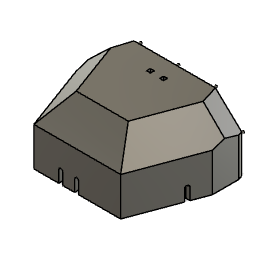
Seismo Case Top S1 v2 (Autodesk Fusion 360 design; units mm, degrees)
Autodesk Fusion 360 part; units mm, degrees
sketch "Sketch1" plane through (0, 0, 0) normal (0, 1, 0) x (1, 0, 0)
  line L0 (-69.1818, 27.2298) -> (-69.1818, -12.7702)
  line L1 (-69.1818, 27.2298) -> (-31.3668, 147.2296)
  line L2 (-31.3668, 147.2296) -> (98.6332, 147.2296)
  line L3 (98.6332, 147.2296) -> (136.3099, 27.1863)
  line L4 (136.3099, 27.1863) -> (136.3099, -12.8137)
  line L5 (136.3099, -12.8137) -> (98.5054, -114.5242)
  line L6 (-69.1818, -12.7702) -> (-31.4946, -114.5242)
  line L7 (-31.4946, -114.5242) -> (98.5054, -114.5242)
  line L8 (-36.0236, 153.5796) -> (103.2956, 153.5796)
  line L9 (103.2956, 153.5796) -> (142.6599, 28.1594)
  line L10 (142.6599, 28.1594) -> (142.6599, -13.9557)
  line L11 (142.6599, -13.9557) -> (102.9196, -120.8742)
  line L12 (102.9196, -120.8742) -> (-35.9143, -120.8742)
  line L13 (-35.9143, -120.8742) -> (-75.5318, -13.9084)
  line L14 (-75.5318, -13.9084) -> (-75.5318, 28.2067)
  line L15 (-75.5318, 28.2067) -> (-36.0236, 153.5796)
  dimension "d1" = 40
  dimension "d2" = 125.817
  dimension "d5" = 125.817
  dimension "d6" = 40
  dimension "d8" = 108.509
  dimension "d10" = 108.509
  dimension "d12" = 162.509
  dimension "d14" = 6.35
  dimension "d15" = 6.35
  dimension "d16" = 6.35
  dimension "d17" = 6.35
  dimension "d18" = 6.35
  dimension "d19" = 6.35
  dimension "d20" = 6.35
  dimension "d21" = 6.35
  dimension "d44" = 130
  dimension "d49" = 130
  constraint vertical L0
  constraint horizontal L2
  constraint vertical L4
  constraint parallel L2 L8
  constraint parallel L3 L9
  constraint perpendicular L8 L10
  constraint parallel L5 L11
  constraint horizontal L12
  constraint vertical L14
  constraint parallel L6 L13
  measures "d1" distance of L0.start L0.end
  measures "d2" distance of L0.start L1.end
  measures "d5" distance of L2.end L3.end
  measures "d6" distance of L3.end L4.end
  measures "d8" distance of L4.end L5.end
  measures "d10" distance of L0.end L6.end
  measures "d12" angle of L14 L15
  measures "d14" distance of L5 L11
  measures "d15" distance of L4 L10
  measures "d16" distance of L3 L9
  measures "d17" distance of L2 L8
  measures "d18" distance of L1 L15
  measures "d19" distance of L0 L14
  measures "d20" distance of L6 L13
  measures "d21" distance of L7 L12
  measures "d44" distance of L1.end L2.end
  measures "d49" distance of L5.end L6.end
extrude "Extrude1" add sketch "Sketch1" along normal blind 101.6 contours L0 L1 L2 L3 L4 L5 L6 L7 | L8 L9 L10 L11 L12 L13 L14 L15 makes body 1
chamfer "Chamfer1" distance 40 angle 45 6 edges at (-55.7231, 101.6, 67.3913) (33.5026, 101.6, 120.8742) (122.7897, 101.6, 67.4149) (122.9777, 101.6, -90.8695) (33.636, 101.6, -153.5796) (-55.7777, 101.6, -90.8931) on bodies 1
shell "Shell1" thickness 6.35 removed faces 1 at (10.3681, 0, -69.9819) on bodies 1
sketch "Sketch2" plane through (0, 0, 0) normal (0, 1, 0) x (1, 0, 0)
  line L0 (-21.4696, -108.1492) -> (-15.1696, -108.1492)
  line L1 (-15.1696, -108.1492) -> (-15.1696, -101.8492)
  line L2 (-15.1696, -101.8492) -> (-21.4696, -101.8492)
  line L3 (-21.4696, -101.8492) -> (-21.4696, -108.1492)
  line L4 (82.1804, -108.1492) -> (88.4804, -108.1492)
  line L5 (88.4804, -108.1492) -> (88.4804, -101.8492)
  line L6 (88.4804, -101.8492) -> (82.1804, -101.8492)
  line L7 (82.1804, -101.8492) -> (82.1804, -108.1492)
  line L8 (-62.8068, -9.899) -> (-56.5068, -9.899)
  line L9 (-56.5068, -9.899) -> (-56.5068, -3.599)
  line L10 (-56.5068, -3.599) -> (-62.8068, -3.599)
  line L11 (-62.8068, -3.599) -> (-62.8068, -9.899)
  line L12 (-56.5068, 17.9048) -> (-62.8068, 17.9048)
  line L13 (-62.8068, 17.9048) -> (-62.8068, 24.2048)
  line L14 (-62.8068, 24.2048) -> (-56.5068, 24.2048)
  line L15 (-56.5068, 24.2048) -> (-56.5068, 17.9048)
  line L16 (-21.3418, 134.5546) -> (-15.0418, 134.5546)
  line L17 (-15.0418, 134.5546) -> (-15.0418, 140.8546)
  line L18 (-15.0418, 140.8546) -> (-21.3418, 140.8546)
  line L19 (-21.3418, 140.8546) -> (-21.3418, 134.5546)
  line L20 (82.3082, 140.8546) -> (88.6082, 140.8546)
  line L21 (88.6082, 140.8546) -> (88.6082, 134.5546)
  line L22 (88.6082, 134.5546) -> (82.3082, 134.5546)
  line L23 (82.3082, 134.5546) -> (82.3082, 140.8546)
  line L24 (129.9349, 17.8613) -> (123.6349, 17.8613)
  line L25 (123.6349, 17.8613) -> (123.6349, 24.1613)
  line L26 (123.6349, 24.1613) -> (129.9349, 24.1613)
  line L27 (129.9349, 24.1613) -> (129.9349, 17.8613)
  line L28 (123.6349, -9.7887) -> (129.9349, -9.7887)
  line L29 (129.9349, -9.7887) -> (129.9349, -3.4887)
  line L30 (129.9349, -3.4887) -> (123.6349, -3.4887)
  line L31 (123.6349, -3.4887) -> (123.6349, -9.7887)
  point P0 (-31.4946, -114.5242)
  point P1 (98.5054, -114.5242)
  point P2 (-69.1818, 27.2298)
  point P3 (98.6332, 147.2296)
  point P4 (-31.3668, 147.2296)
  point P5 (136.3099, 27.1863)
  point P6 (136.3099, -12.8137)
  dimension "d26" = 6.3
  dimension "d27" = 6.3
  dimension "d28" = 6.3
  dimension "d29" = 6.3
  dimension "d34" = 6.3
  dimension "d35" = 6.3
  dimension "d36" = 6.3
  dimension "d37" = 6.3
  dimension "d50" = 10.025
  dimension "d51" = 6.375
  dimension "d52" = 10.025
  dimension "d53" = 6.375
  dimension "d54" = 3.025
  dimension "d55" = 6.375
  dimension "d57" = 6.3
  dimension "d58" = 6.3
  dimension "d59" = 6.3
  dimension "d60" = 6.3
  dimension "d61" = 10.025
  dimension "d62" = 10.025
  dimension "d63" = 6.375
  dimension "d64" = 6.375
  dimension "d65" = 6.3
  dimension "d66" = 6.3
  dimension "d67" = 6.375
  dimension "d68" = 3.025
  dimension "d69" = 6.3
  dimension "d70" = 6.3
  dimension "d71" = 3.025
  dimension "d72" = 6.375
  dimension "d95" = 6.375
  constraint horizontal L0
  constraint vertical L1
  constraint horizontal L2
  constraint vertical L3
  constraint horizontal L4
  constraint vertical L5
  constraint horizontal L6
  constraint vertical L7
  constraint horizontal L8
  constraint vertical L9
  constraint horizontal L10
  constraint vertical L11
  constraint horizontal L12
  constraint vertical L13
  constraint horizontal L14
  constraint vertical L15
  constraint horizontal L16
  constraint vertical L17
  constraint horizontal L18
  constraint vertical L19
  constraint horizontal L20
  constraint vertical L21
  constraint horizontal L22
  constraint vertical L23
  constraint horizontal L24
  constraint vertical L25
  constraint horizontal L26
  constraint vertical L27
  constraint horizontal L28
  constraint vertical L29
  constraint horizontal L30
  constraint vertical L31
  measures "d26" distance of L0.end L1.end
  measures "d27" distance of L1.end L2.end
  measures "d28" distance of L4.start L6.end
  measures "d29" distance of L5.end L6.end
  measures "d34" distance of L8.start L10.end
  measures "d35" distance of L8.start L8.end
  measures "d36" distance of L12.start L14.end
  measures "d37" distance of L12.start L12.end
  measures "d50" horizontal distance of L2.end P0
  measures "d51" distance of L0 P0
  measures "d52" horizontal distance of L4.end P1
  measures "d53" vertical distance of L4.end P1
  measures "d54" vertical distance of L14.end P2
  measures "d55" distance of L13 P2
  measures "d57" distance of L16.start L16.end
  measures "d58" distance of L16.start L18.end
  measures "d59" distance of L20.start L22.end
  measures "d60" distance of L21.end L22.end
  measures "d61" horizontal distance of L21.end P3
  measures "d62" horizontal distance of L18.end P4
  measures "d63" distance of L18 P4
  measures "d64" distance of L20 P3
  measures "d65" distance of L24.start L24.end
  measures "d66" distance of L24.end L25.end
  measures "d67" horizontal distance of L26.end P5
  measures "d68" vertical distance of L26.end P5
  measures "d69" distance of L28.start L28.end
  measures "d70" distance of L28.start L30.end
  measures "d71" vertical distance of L28.end P6
  measures "d72" horizontal distance of L28.end P6
  measures "d95" distance of L11 P2
extrude "Extrude2" add sketch "Sketch2" along normal blind 12.7 separate body makes body 2 at (-21.3418, 4.2333, -138.7546) makes body 3 at (86.3804, 8.4667, 101.8492) makes body 4 at (127.8349, 4.2333, 3.4887) makes body 5 at (-58.6068, 4.2333, -17.9048) makes body 6 at (84.4082, 8.4667, -140.8546) makes body 7 at (-21.4696, 4.2333, 103.9492) makes body 8 at (127.8349, 4.2333, -17.8613) makes body 9 at (-62.8068, 8.4667, 5.699)
sketch "Sketch3" plane through (0, 0, -24.1613) normal (0, 0, -1) x (-1, 0, 0)
  line L0 (-129.9349, 0) -> (-123.6349, 0)
  line L1 (-123.6349, 0) -> (-123.6349, 12.7)
  line L2 (-123.6349, 12.7) -> (-129.9349, 12.7)
  line L3 (-129.9349, 12.7) -> (-129.9349, 0)
  line L4 (-123.6349, 12.7) -> (-123.6349, 17.7)
  line L5 (-129.9349, 12.7) -> (-136.3099, 16.7476)
  line L6 (-123.6349, 17.7) -> (-136.3099, 25.7476)
  line L7 (-136.3099, 25.7476) -> (-136.3099, 16.7476)
  dimension "d75" = 5
  dimension "d76" = 6.375
  dimension "d80" = 9
  constraint coincident L1.end L2.start
  constraint perpendicular L2 L4
  constraint coincident L2.end L3.start
  constraint parallel L4 L7
  constraint parallel L5 L6
  measures "d75" distance of L1.end L4.end
  measures "d76" horizontal distance of L2.end L5.end
  measures "d80" distance of L5.end L6.end
extrude "Extrude3" add sketch "Sketch3" against normal blind 33.95 contours L2 L4 L5 L6 L7 bodies 4 8
sketch "Sketch4" plane through (88.4804, 0, 0) normal (1, 0, 0) x (0, 0, -1)
  line L0 (-108.1492, 0) -> (-101.8492, 0)
  line L1 (-101.8492, 0) -> (-101.8492, 12.7)
  line L2 (-101.8492, 12.7) -> (-108.1492, 12.7)
  line L3 (-108.1492, 12.7) -> (-108.1492, 0)
  line L4 (-101.8492, 12.7) -> (-101.8492, 17.7)
  line L5 (-101.8492, 17.7) -> (-114.5242, 25.7476)
  line L6 (-114.5242, 25.7476) -> (-114.5242, 16.7476)
  line L7 (-114.5242, 16.7476) -> (-108.1492, 12.7)
  dimension "d79" = 6.375
  dimension "d81" = 5
  dimension "d82" = 9
  constraint coincident L1.end L2.start
  constraint perpendicular L2 L4
  constraint perpendicular L2 L6
  constraint coincident L2.end L3.start
  constraint parallel L5 L7
  measures "d79" horizontal distance of L6.end L2.end
  measures "d81" distance of L1.end L4.end
  measures "d82" distance of L5.end L6.end
extrude "Extrude4" add sketch "Sketch4" against normal blind 109.95 contours L2 L4 L5 L6 L7 bodies 3 7
sketch "Sketch5" plane through (-21.3418, 0, 0) normal (-1, 0, 0) x (0, 0, 1)
  line L0 (-140.8546, 0) -> (-134.5546, 0)
  line L1 (-134.5546, 0) -> (-134.5546, 12.7)
  line L2 (-134.5546, 12.7) -> (-140.8546, 12.7)
  line L3 (-140.8546, 12.7) -> (-140.8546, 0)
  line L4 (-134.5546, 12.7) -> (-134.5546, 17.7)
  line L5 (-134.5546, 17.7) -> (-147.2296, 25.7476)
  line L6 (-147.2296, 25.7476) -> (-147.2296, 16.7476)
  line L7 (-147.2296, 16.7476) -> (-140.8546, 12.7)
  dimension "d85" = 5
  dimension "d86" = 9
  dimension "d87" = 6.375
  constraint coincident L1.end L2.start
  constraint perpendicular L2 L4
  constraint parallel L4 L6
  constraint coincident L2.end L3.start
  constraint parallel L5 L7
  measures "d85" distance of L1.end L4.end
  measures "d86" distance of L5.end L6.end
  measures "d87" horizontal distance of L6.end L2.end
extrude "Extrude5" add sketch "Sketch5" against normal blind 109.95 contours L2 L4 L5 L6 L7 bodies 2 6
sketch "Sketch6" plane through (0, 0, 9.899) normal (0, 0, 1) x (1, 0, 0)
  line L0 (-62.8068, 0) -> (-56.5068, 0)
  line L1 (-56.5068, 0) -> (-56.5068, 12.7)
  line L2 (-56.5068, 12.7) -> (-62.8068, 12.7)
  line L3 (-62.8068, 12.7) -> (-62.8068, 0)
  line L4 (-56.5068, 12.7) -> (-56.5068, 17.7)
  line L5 (-56.5068, 17.7) -> (-69.1818, 25.7476)
  line L6 (-69.1818, 25.7476) -> (-69.1818, 16.7476)
  line L7 (-69.1818, 16.7476) -> (-62.8068, 12.7)
  dimension "d90" = 6.375
  dimension "d91" = 5
  dimension "d92" = 9
  constraint coincident L1.end L2.start
  constraint perpendicular L2 L4
  constraint parallel L4 L6
  constraint coincident L2.end L3.start
  constraint parallel L5 L7
  measures "d90" horizontal distance of L6.end L2.end
  measures "d91" distance of L1.end L4.end
  measures "d92" distance of L5.end L6.end
extrude "Extrude6" add sketch "Sketch6" against normal blind 34.104 contours L2 L4 L5 L6 L7 bodies 5 9
sketch "Sketch7" plane through (0, 95.25, 0) normal (0, -1, 0) x (1, 0, 0)
  line L0 (-37.6546, -6.5657) -> (-4.7606, -110.9493)
  line L1 (-4.7606, -110.9493) -> (71.9949, -110.9493)
  line L2 (71.9949, -110.9493) -> (104.78, -6.4912)
  line L3 (104.78, -6.4912) -> (73.285, 78.2439)
  line L4 (73.285, 78.2439) -> (-6.2432, 78.2439)
  line L5 (-6.2432, 78.2439) -> (-37.6546, -6.5657)
  line L6 (11.3454, 13.2439) -> (55.7954, 13.2439)
  line L7 (55.7954, 13.2439) -> (55.7954, -28.6661)
  line L8 (55.7954, -28.6661) -> (11.3454, -28.6661)
  line L9 (11.3454, -28.6661) -> (11.3454, 13.2439)
  dimension "d96" = 44.45
  dimension "d97" = 41.91
  dimension "d98" = 65
  dimension "d99" = 49
  constraint horizontal L6
  constraint vertical L7
  constraint horizontal L8
  constraint vertical L9
  measures "d96" distance of L6.start L6.end
  measures "d97" distance of L6.end L7.end
  measures "d98" distance of L3.end L6
  measures "d99" distance of L0.start L9
extrude "Extrude7" add sketch "Sketch7" along normal blind 38.1 contours L6 L7 L8 L9 bodies 1
sketch "Sketch8" plane through (0, 0, 13.2439) normal (0, 0, 1) x (1, 0, 0)
  line L0 (55.7954, 95.25) -> (11.3454, 95.25)
  line L1 (11.3454, 95.25) -> (11.3454, 57.15)
  line L2 (11.3454, 57.15) -> (55.7954, 57.15)
  line L3 (55.7954, 57.15) -> (55.7954, 95.25)
  line L4 (49.4454, 63.5) -> (17.6954, 63.5)
  line L5 (17.6954, 63.5) -> (17.6954, 95.125)
  line L6 (17.6954, 95.125) -> (49.4454, 95.125)
  line L7 (49.4454, 95.125) -> (49.4454, 63.5)
  dimension "d102" = 6.35
  dimension "d103" = 6.35
  dimension "d104" = 6.35
  dimension "d105" = 0.125
  constraint horizontal L4
  constraint vertical L5
  constraint horizontal L6
  constraint vertical L7
  measures "d102" distance of L3 L7
  measures "d103" distance of L1 L5
  measures "d104" distance of L2 L4
  measures "d105" distance of L0 L6
extrude "Extrude8" cut sketch "Sketch8" against normal blind 55 contours L4 L5 L6 L7 bodies 1
sketch "Sketch9" plane through (11.3454, 0, 0) normal (-1, 0, 0) x (0, 0, 1)
  line L0 (13.2439, 95.25) -> (-28.6661, 95.25)
  line L1 (-28.6661, 95.25) -> (-28.6661, 57.15)
  line L2 (-28.6661, 57.15) -> (13.2439, 57.15)
  line L3 (13.2439, 57.15) -> (13.2439, 95.25)
  line L4 (-22.3161, 95.125) -> (6.8939, 95.125)
  line L5 (6.8939, 95.125) -> (6.8939, 63.5)
  line L6 (6.8939, 63.5) -> (-22.3161, 63.5)
  line L7 (-22.3161, 63.5) -> (-22.3161, 95.125)
  dimension "d108" = 6.35
  dimension "d109" = 6.35
  dimension "d110" = 6.35
  dimension "d111" = 0.125
  constraint horizontal L4
  constraint vertical L5
  constraint horizontal L6
  constraint vertical L7
  measures "d108" distance of L1 L7
  measures "d109" distance of L3 L5
  measures "d110" distance of L2 L6
  measures "d111" distance of L0 L4
extrude "Extrude9" cut sketch "Sketch9" against normal blind 50 contours L4 L5 L6 L7 bodies 1
sketch "Sketch10" plane through (0, 57.15, 0) normal (0, -1, 0) x (1, 0, 0)
  line L0 (11.3454, -28.6661) -> (55.7954, -28.6661)
  line L1 (55.7954, -28.6661) -> (55.7954, 13.2439)
  line L2 (55.7954, 13.2439) -> (11.3454, 13.2439)
  line L3 (11.3454, 13.2439) -> (11.3454, -28.6661)
  line L4 (14.5204, 10.0689) -> (52.6204, 10.0689)
  line L5 (52.6204, 10.0689) -> (52.6204, -25.4911)
  line L6 (52.6204, -25.4911) -> (14.5204, -25.4911)
  line L7 (14.5204, -25.4911) -> (14.5204, 10.0689)
  dimension "d120" = 38.1
  dimension "d121" = 35.56
  dimension "d122" = 3.175
  dimension "d123" = 3.175
  dimension "d124" = 3.175
  constraint horizontal L4
  constraint vertical L5
  constraint horizontal L6
  constraint vertical L7
  measures "d120" distance of L4.start L4.end
  measures "d121" distance of L4.end L5.end
  measures "d122" distance of L1 L5
  measures "d123" distance of L2 L4
  measures "d124" distance of L0 L6
extrude "Extrude10" cut sketch "Sketch10" against normal blind 38.1 contours L4 L5 L6 L7 bodies 1
sketch "Sketch11" plane through (0, 57.15, 0) normal (0, -1, 0) x (1, 0, 0)
  line L0 (52.6204, 10.0689) -> (52.6204, -25.4911)
  line L1 (52.6204, -25.4911) -> (14.5204, -25.4911)
  line L2 (14.5204, -25.4911) -> (14.5204, 10.0689)
  line L3 (14.5204, 10.0689) -> (52.6204, 10.0689)
  line L4 (11.3454, -28.6661) -> (55.7954, -28.6661)
  line L5 (55.7954, -28.6661) -> (55.7954, 13.2439)
  line L6 (55.7954, 13.2439) -> (11.3454, 13.2439)
  line L7 (11.3454, 13.2439) -> (11.3454, -28.6661)
  line L8 (14.5204, 10.0689) -> (52.6204, 10.0689)
  line L9 (52.6204, 10.0689) -> (52.6204, -25.4911)
  line L10 (52.6204, -25.4911) -> (14.5204, -25.4911)
  line L11 (14.5204, -25.4911) -> (14.5204, 10.0689)
  line L12 (17.0604, 7.5289) -> (50.0804, 7.5289)
  line L13 (50.0804, 7.5289) -> (50.0804, -22.9511)
  line L14 (50.0804, -22.9511) -> (17.0604, -22.9511)
  line L15 (17.0604, -22.9511) -> (17.0604, 7.5289)
  dimension "d125" = 2.54
  dimension "d126" = 2.54
  dimension "d127" = 2.54
  dimension "d128" = 2.54
  constraint horizontal L8
  constraint vertical L9
  constraint horizontal L10
  constraint vertical L11
  constraint coincident L0.end L1.start
  constraint coincident L2.end L3.start
  constraint horizontal L12
  constraint vertical L13
  constraint horizontal L14
  constraint vertical L15
  measures "d125" distance of L9 L13
  measures "d126" distance of L8 L12
  measures "d127" distance of L11 L15
  measures "d128" distance of L10 L14
extrude "Extrude11" add sketch "Sketch11" against normal blind 6.35 contours L0 L1 L2 L3 L8 L9 L10 L11 bodies 1
sketch "Sketch12" plane through (0, 95.25, 0) normal (0, -1, 0) x (1, 0, 0)
  line L0 (14.5204, -25.4911) -> (52.6204, -25.4911)
  line L1 (52.6204, -25.4911) -> (52.6204, 10.0689)
  line L2 (52.6204, 10.0689) -> (14.5204, 10.0689)
  line L3 (14.5204, 10.0689) -> (14.5204, -25.4911)
  line L4 (19.9704, -3.5177) -> (26.0664, -3.5177)
  line L5 (26.0664, -3.5177) -> (26.0664, -9.6137)
  line L6 (26.0664, -9.6137) -> (19.9704, -9.6137)
  line L7 (19.9704, -9.6137) -> (19.9704, -3.5177)
  line L8 (41.0664, -3.4432) -> (47.1624, -3.4432)
  line L9 (47.1624, -3.4432) -> (47.1624, -9.5392)
  line L10 (47.1624, -9.5392) -> (41.0664, -9.5392)
  line L11 (41.0664, -9.5392) -> (41.0664, -3.4432)
  point P0 (-37.6546, -6.5657)
  point P1 (104.78, -6.4912)
  dimension "d131" = 6.096
  dimension "d132" = 6.096
  dimension "d133" = 6.096
  dimension "d134" = 6.096
  dimension "d135" = 3.048
  dimension "d136" = 3.048
  dimension "d137" = 15
  dimension "d138" = 5.45
  constraint horizontal L4
  constraint vertical L5
  constraint horizontal L6
  constraint vertical L7
  constraint horizontal L8
  constraint vertical L9
  constraint horizontal L10
  constraint vertical L11
  measures "d131" distance of L4.start L6.end
  measures "d132" distance of L4.start L4.end
  measures "d133" distance of L8.start L8.end
  measures "d134" distance of L8.end L9.end
  measures "d135" vertical distance of L4.start P0
  measures "d136" vertical distance of L9.end P1
  measures "d137" distance of L5 L11
  measures "d138" distance of L3 L7
extrude "Extrude12" cut sketch "Sketch12" against normal blind 70 contours L4 L5 L6 L7 | L8 L9 L10 L11 bodies 1
sketch "Sketch13" plane through (0, 0, 120.8742) normal (0, 0, 1) x (1, 0, 0)
  line L0 (102.9196, 61.6) -> (-35.9143, 61.6)
  line L1 (-35.9143, 61.6) -> (-35.9143, 0)
  line L2 (-35.9143, 0) -> (102.9196, 0)
  line L3 (102.9196, 0) -> (102.9196, 61.6)
  line L4 (3.8804, 0) -> (10.2304, 0)
  line L5 (10.2304, 0) -> (10.2304, 19.05)
  line L6 (10.2304, 19.05) -> (3.8804, 19.05)
  line L7 (3.8804, 19.05) -> (3.8804, 0)
  arc A0 (10.2304, 19.05) -> (3.8804, 19.05) centre (7.0554, 19.05) ccw
  line L8 (29.2804, 0) -> (35.6304, 0)
  line L9 (35.6304, 0) -> (35.6304, 19.05)
  line L10 (35.6304, 19.05) -> (29.2804, 19.05)
  line L11 (29.2804, 19.05) -> (29.2804, 0)
  arc A1 (35.6304, 19.05) -> (29.2804, 19.05) centre (32.4554, 19.05) ccw
  point P0 (-15.1696, 0)
  dimension "d141" = 6.35
  dimension "d142" = 19.05
  dimension "d143" = 19.05
  dimension "d144" = 19.05
  dimension "d145" = 19.05
  dimension "d146" = 6.35
  constraint horizontal L4
  constraint vertical L5
  constraint horizontal L6
  constraint vertical L7
  constraint coincident L2 L4.start
  constraint tangent L5 A0
  constraint horizontal L8
  constraint vertical L9
  constraint horizontal L10
  constraint vertical L11
  constraint coincident L2 L8.start
  constraint tangent L9 A1
  measures "d141" distance of L4.start L4.end
  measures "d142" distance of L4.start P0
  measures "d143" distance of L4.end L5.end
  measures "d144" distance of L8.end L9.end
  measures "d145" distance of L5 L11
  measures "d146" distance of L8.start L8.end
extrude "Extrude13" cut sketch "Sketch13" against normal blind 6.35 contours L2 L8 L9 L10 L11 | L2 L4 L5 L6 L7 | L10 A1 | L6 A0 bodies 1
sketch "Sketch14" plane through (142.6599, 0, 0) normal (1, 0, 0) x (0, 0, -1)
  line L0 (28.1594, 61.6) -> (5.511, 68.3822)
  line L1 (5.511, 68.3822) -> (-13.9557, 61.6)
  line L2 (-13.9557, 61.6) -> (-13.9557, 0)
  line L3 (-13.9557, 0) -> (28.1594, 0)
  line L4 (28.1594, 0) -> (28.1594, 61.6)
  line L5 (81.3344, 0) -> (87.6844, 0)
  line L6 (87.6844, 0) -> (87.6844, 19.05)
  line L7 (87.6844, 19.05) -> (81.3344, 19.05)
  line L8 (81.3344, 19.05) -> (81.3344, 0)
  arc A0 (87.6844, 19.05) -> (81.3344, 19.05) centre (84.5094, 19.05) ccw
  line L9 (-39.9557, 0) -> (-46.3057, 0)
  line L10 (-46.3057, 0) -> (-46.3057, 19.05)
  line L11 (-46.3057, 19.05) -> (-39.9557, 19.05)
  line L12 (-39.9557, 19.05) -> (-39.9557, 0)
  arc A1 (-39.9557, 19.05) -> (-46.3057, 19.05) centre (-43.1307, 19.05) ccw
  dimension "d149" = 53.175
  dimension "d150" = 6.35
  dimension "d151" = 19.05
  dimension "d152" = 6.35
  dimension "d153" = 19.05
  dimension "d154" = 26
  constraint horizontal L5
  constraint vertical L6
  constraint horizontal L7
  constraint vertical L8
  constraint tangent L6 A0
  constraint horizontal L9
  constraint vertical L10
  constraint horizontal L11
  constraint vertical L12
  constraint tangent L12 A1
  measures "d149" distance of L3.end L5.start
  measures "d150" distance of L5.start L5.end
  measures "d151" distance of L5.end L6.end
  measures "d152" distance of L9.start L9.end
  measures "d153" distance of L9.start L11.end
  measures "d154" distance of L2.end L9.start
extrude "Extrude14" cut sketch "Sketch14" against normal blind 30 contours L5 L6 L7 L8 | L7 A0 | L9 L10 L11 L12 | L11 A1 bodies 1
sketch "Sketch15" plane through (0, 0, 0) normal (0, -1, 0) x (1, 0, 0)
  line L0 (123.9774, -87.6844) -> (117.322, -87.6844)
  line L1 (117.322, -87.6844) -> (98.6332, -147.2296)
  line L2 (98.6332, -147.2296) -> (-31.3668, -147.2296)
  line L3 (-31.3668, -147.2296) -> (-69.1818, -27.2298)
  line L4 (-69.1818, -27.2298) -> (-69.1818, 12.7702)
  line L5 (-69.1818, 12.7702) -> (-31.4946, 114.5242)
  line L6 (-31.4946, 114.5242) -> (3.8804, 114.5242)
  line L7 (3.8804, 114.5242) -> (3.8804, 120.8742)
  line L8 (3.8804, 120.8742) -> (-35.9143, 120.8742)
  line L9 (-35.9143, 120.8742) -> (-75.5318, 13.9084)
  line L10 (-75.5318, 13.9084) -> (-75.5318, -28.2067)
  line L11 (-75.5318, -28.2067) -> (-36.0236, -153.5796)
  line L12 (-36.0236, -153.5796) -> (103.2956, -153.5796)
  line L13 (103.2956, -153.5796) -> (123.9774, -87.6844)
  line L14 (155.8182, -34.9634) -> (-94.1818, -34.9634)
  line L15 (-94.1818, -34.9634) -> (-94.1818, -162.4295)
  line L16 (-94.1818, -162.4295) -> (155.8182, -162.4295)
  line L17 (155.8182, -162.4295) -> (155.8182, -34.9634)
  dimension "d157" = 250
  dimension "d159" = 25
  constraint horizontal L14
  constraint vertical L15
  constraint horizontal L16
  constraint vertical L17
  measures "d157" distance of L15.end L16.end
  measures "d159" distance of L4 L15
extrude "Extrude15" cut sketch "Sketch15" against normal blind 120 contours L0 L1 L2 L3 L11 L12 L13 L14 | L0 L1 L2 L3 L11 L12 L13 L14 L15 L16 L17 bodies 1 2
sketch "Sketch16" plane through (0, 0, -34.9634) normal (0, 0, -1) x (-1, 0, 0)
  line L0 (73.4026, 0) -> (73.4026, 61.6)
  line L1 (73.4026, 61.6) -> (31.4635, 101.6)
  line L2 (31.4635, 101.6) -> (-98.6005, 101.6)
  line L3 (-98.6005, 101.6) -> (-140.5244, 61.6)
  line L4 (-140.5244, 61.6) -> (-140.5244, 0)
  line L5 (-140.5244, 0) -> (-133.8689, 0)
  line L6 (-133.8689, 0) -> (-133.8689, 58.9697)
  line L7 (-133.8689, 58.9697) -> (-95.8437, 95.25)
  line L8 (-95.8437, 95.25) -> (28.7058, 95.25)
  line L9 (28.7058, 95.25) -> (66.7448, 58.9697)
  line L10 (66.7448, 58.9697) -> (66.7448, 0)
  line L11 (66.7448, 0) -> (73.4026, 0)
  circle A0 centre (-33.569, 98.425) radius 1.5875
  circle A1 centre (-93.6005, 98.425) radius 1.5875
  circle A2 centre (26.4635, 98.425) radius 1.5875
  circle A3 centre (-137.3494, 56.6) radius 1.5875
  circle A4 centre (70.2276, 56.6) radius 1.5875
  dimension "d162" = 3.175
  dimension "d163" = 3.175
  dimension "d164" = 65.0315
  dimension "d165" = 3.175
  dimension "d166" = 3.175
  dimension "d167" = 5
  dimension "d168" = 3.175
  dimension "d169" = 3.175
  dimension "d170" = 5
  dimension "d171" = 3.175
  dimension "d172" = 3.175
  dimension "d173" = 5
  dimension "d174" = 3.175
  dimension "d176" = 5
  dimension "d177" = 3.175
  measures "d162" diameter of A0
  measures "d163" distance of L2 A0.centre
  measures "d164" horizontal distance of L2.end A0.centre
  measures "d165" diameter of A1
  measures "d166" distance of L2 A1.centre
  measures "d167" horizontal distance of L2.end A1.centre
  measures "d168" diameter of A2
  measures "d169" distance of L2 A2.centre
  measures "d170" horizontal distance of L1.end A2.centre
  measures "d171" diameter of A3
  measures "d172" distance of L4 A3.centre
  measures "d173" vertical distance of L3.end A3.centre
  measures "d174" diameter of A4
  measures "d176" vertical distance of L0.end A4.centre
  measures "d177" distance of L0 A4.centre
extrude "Extrude16" add sketch "Sketch16" along normal blind 6.35 contours A0 | A1 | A2 | A3 | A4 bodies 1 2
equation "d10 = d8"
